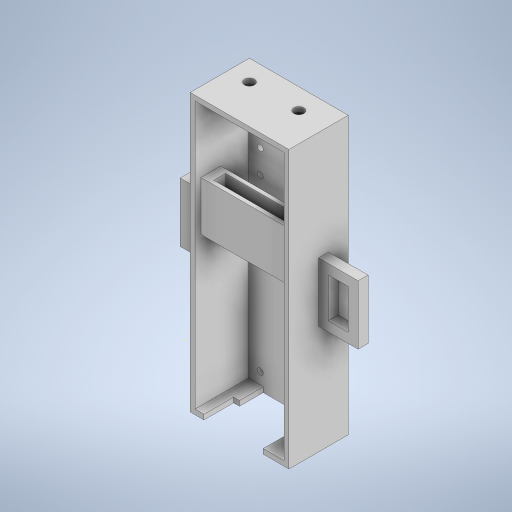
# Autodesk Inventor part: arduino mould_3r
Saved by Autodesk Inventor 2023 (Build 270158000, 158)
## iProperties
Created: 2023-05-04
Part Number: arduino mould_3r
Material: Generic
Document SubType Name: Modeling
Designer: gmami
Density: 1 g/cm^3
Appearance: Default
Author: gmami
Autodesk Inventor part; units mm, degrees
ref_plane "YZ Plane" through (0, 0, 0) normal (1, 0, 0) x (0, 1, 0)
sketch "Sketch1" plane through (0, 0, 0) normal (0, 0, 1) x (1, 0, 0)
  line L0 (33.3378, 145.104) -> (83.3378, 145.104)
  line L1 (83.3378, 145.104) -> (83.3378, 5.104)
  line L2 (83.3378, 5.104) -> (33.3378, 5.104)
  line L3 (33.3378, 5.104) -> (33.3378, 145.104)
  line L4 (33.3378, 90.104) -> (33.3378, 60.104)
  line L5 (83.3378, 90.104) -> (83.3378, 60.104)
  point P0 (0, 0)
  dimension "d0" = 140
  dimension "d1" = 50
  constraints: 12 end point, 2 parallel, 2 point on line, 1 horizontal, 1 perpendicular
  measures "d0" distance of L2.end L0.start
  measures "d1" distance of L1.end L2.end
extrude "Extrusion1" add sketch "Sketch1" along normal blind 30
sketch "Sketch2" plane through (0, 0, 30) normal (0, 0, 1) x (1, 0, 0)
  line L0 (35.8378, 142.604) -> (80.8378, 142.604)
  line L1 (80.8378, 142.604) -> (80.8378, 7.604)
  line L2 (80.8378, 7.604) -> (35.8378, 7.604)
  line L3 (35.8378, 7.604) -> (35.8378, 142.604)
  line L4 (83.3378, 145.104) -> (33.3378, 145.104) projected
  line L5 (83.3378, 5.104) -> (83.3378, 145.104) projected
  line L6 (33.3378, 5.104) -> (83.3378, 5.104) projected
  line L7 (33.3378, 145.104) -> (33.3378, 5.104) projected
  point P0 (0, 0)
  point P1 (58.3378, 142.604)
  dimension "d4" = 2.5
  dimension "d5" = 2.5
  dimension "d6" = 2.5
  dimension "d7" = 2.5
  constraints: 8 end point, 2 parallel, 1 horizontal, 1 midpoint, 1 perpendicular
  measures "d4" distance from line of L4 point (58.338, 142.604)
  measures "d5" distance between parallel lines of L5 L1
  measures "d6" distance between parallel lines of L2 L6
  measures "d7" distance between parallel lines of L3 L7
extrude "Extrusion2" cut sketch "Sketch2" against normal blind 27 contours L0 L1 L2 L3
sketch "Sketch3" plane through (33.3378, 5.104, 0) normal (0, -1, 0) x (1, 0, 0)
  line L0 (7, 30) -> (37, 30)
  line L1 (37, 30) -> (37, 15)
  line L2 (37, 15) -> (7, 15)
  line L3 (7, 15) -> (7, 30)
  line L4 (0, 0) -> (50, 0) projected
  line L5 (0, 0) -> (0, 30) projected
  line L6 (0, 30) -> (50, 30) projected
  line L7 (10, 15) -> (35, 15)
  line L8 (35, 15) -> (35, 3)
  line L9 (35, 3) -> (10, 3)
  line L10 (10, 3) -> (10, 15)
  point P0 (-33.3378, 0)
  point P1 (37, 22.5)
  point P2 (10, 9)
  dimension "d10" = 15
  dimension "d11" = 30
  dimension "d12" = 7
  dimension "d13" = 0
  dimension "d14" = 25
  dimension "d15" = 10
  dimension "d16" = 3
  constraints: 16 end point, 4 parallel, 2 horizontal, 2 midpoint, 2 perpendicular, 1 point on line
  measures "d10" distance between parallel lines of L2 L4
  measures "d11" distance from line of point (37, 22.5) L3
  measures "d12" distance between parallel lines of L3 L5
  measures "d13" distance between parallel lines of L6 L0
  measures "d14" distance between parallel lines of L8 L10
  measures "d15" distance from line of L5 point (10, 9)
  measures "d16" distance between parallel lines of L4 L9
extrude "Extrusion3" cut sketch "Sketch3" against normal blind 27
sketch "Sketch4" plane through (0, 0, 0) normal (0, 0, -1) x (-1, 0, 0)
  circle A0 centre (-74.8378, 13.604) radius 1.5
  circle A1 centre (-41.8378, 13.604) radius 1.5
  circle A2 centre (-41.8378, 99.604) radius 1.5
  circle A3 centre (-74.8378, 99.604) radius 1.5
  circle A4 centre (-41.8378, 111.604) radius 1.5
  circle A5 centre (-74.8378, 111.604) radius 1.5
  line L0 (-83.3378, 5.104) -> (-83.3378, 145.104) projected
  line L1 (-33.3378, 145.104) -> (-33.3378, 5.104) projected
  line L2 (-33.3378, 5.104) -> (-83.3378, 5.104) projected
  line L3 (-83.3378, 145.104) -> (-33.3378, 145.104) projected
  point P0 (0, 0)
  dimension "d19" = 8.5
  dimension "d20" = 8.5
  dimension "d21" = 8.5
  dimension "d22" = 8.5
  dimension "d23" = 3
  dimension "d24" = 3
  dimension "d25" = 8.5
  dimension "d26" = 8.5
  dimension "d27" = 8.5
  dimension "d28" = 8.5
  dimension "d29" = 3
  dimension "d30" = 3
  dimension "d31" = 3
  dimension "d32" = 3
  dimension "d33" = 12
  dimension "d34" = 12
  dimension "d35" = 33.5
  dimension "d36" = 33.5
  constraints: 6 centre point
  measures "d19" distance from line of A0.centre L0
  measures "d20" distance from line of L1 A1.centre
  measures "d21" distance from line of L2 A0.centre
  measures "d22" distance from line of L2 A1.centre
  measures "d23" diameter of A0
  measures "d24" diameter of A1
  measures "d25" distance from line of L1 A2.centre
  measures "d26" distance from line of L1 A4.centre
  measures "d27" distance from line of L0 A5.centre
  measures "d28" distance from line of L0 A3.centre
  measures "d29" diameter of A5
  measures "d30" diameter of A4
  measures "d31" diameter of A2
  measures "d32" diameter of A3
  measures "d33" distance of A3.centre A5.centre
  measures "d34" distance of A2.centre A4.centre
  measures "d35" distance from line of L3 A5.centre
  measures "d36" distance from line of L3 A4.centre
extrude "Extrusion4" cut sketch "Sketch4" against normal blind 27 contours A0 | A1 | A2 | A3 | A4 | A5
sketch "Sketch5" plane through (33.3378, 145.104, 0) normal (0, 1, 0) x (1, 0, 0)
  circle A0 centre (35.5, -10.5) radius 2.5
  circle A1 centre (10.5, -10.5) radius 2.5
  line L0 (50, 0) -> (50, -30) projected
  line L1 (50, 0) -> (0, 0) projected
  point P0 (-33.3378, 0)
  dimension "d39" = 5
  dimension "d40" = 5
  dimension "d41" = 25
  dimension "d42" = 14.5
  dimension "d43" = 10.5
  dimension "d44" = 10.5
  constraints: 2 centre point
  measures "d39" diameter of A0
  measures "d40" diameter of A1
  measures "d41" distance of A1.centre A0.centre
  measures "d42" distance from line of L0 A0.centre
  measures "d43" distance from line of L1 A0.centre
  measures "d44" distance from line of L1 A1.centre
extrude "Extrusion5" cut sketch "Sketch5" against normal blind 27
sketch "Sketch6" plane through (33.3378, 5.104, 0) normal (0, -1, 0) x (1, 0, 0)
  point P0 (-33.3378, 0)
ref_plane "Work Plane1" through (0, 0, 12.5) normal (0, 0, -1) x (-1, 0, 0)
sketch "Sketch7" plane through (0, 0, 12.5) normal (0, 0, -1) x (-1, 0, 0)
  line L0 (-83.3378, 5.104) -> (-83.3378, 145.104) projected
  line L1 (-83.3378, 90.104) -> (-103.3378, 90.104)
  line L2 (-103.3378, 90.104) -> (-103.3378, 60.104)
  line L3 (-103.3378, 60.104) -> (-83.3378, 60.104)
  line L4 (-83.3378, 60.104) -> (-83.3378, 90.104)
  line L5 (-83.3378, 145.104) -> (-33.3378, 145.104) projected
  line L6 (-88.3378, 65.104) -> (-98.3378, 65.104)
  line L7 (-98.3378, 65.104) -> (-98.3378, 85.104)
  line L8 (-98.3378, 85.104) -> (-88.3378, 85.104)
  line L9 (-88.3378, 85.104) -> (-88.3378, 65.104)
  line L10 (-33.3378, 145.104) -> (-33.3378, 5.104) projected
  line L11 (-13.3378, 90.104) -> (-33.3378, 90.104)
  line L12 (-33.3378, 90.104) -> (-33.3378, 60.104)
  line L13 (-33.3378, 60.104) -> (-13.3378, 60.104)
  line L14 (-13.3378, 60.104) -> (-13.3378, 90.104)
  line L15 (-18.3378, 85.104) -> (-28.3378, 85.104)
  line L16 (-28.3378, 85.104) -> (-28.3378, 65.104)
  line L17 (-28.3378, 65.104) -> (-18.3378, 65.104)
  line L18 (-18.3378, 65.104) -> (-18.3378, 85.104)
  point P0 (0, 0)
  point P1 (-93.3378, 60.104)
  dimension "d56" = 20
  dimension "d57" = 30
  dimension "d58" = 55
  dimension "d59" = 5
  dimension "d60" = 20
  dimension "d61" = 30
  dimension "d62" = 55
  dimension "d63" = 5
  constraints: 32 end point, 8 parallel, 4 perpendicular, 2 horizontal, 2 point on line, 1 midpoint, 6 other
  measures "d56" distance between parallel lines of L0 L2
  measures "d57" distance from line of L1 point (-93.338, 60.104)
  measures "d58" distance between parallel lines of L5 L1
  measures "d59" distance between parallel lines of L3 L6
  measures "d60" distance between parallel lines of L12 L14
  measures "d61" distance between parallel lines of L11 L13
  measures "d62" distance between parallel lines of L5 L11
  measures "d63" distance between parallel lines of L14 L18
extrude "Extrusion6" add sketch "Sketch7" along normal mid plane 5
ref_plane "Work Plane2" through (0, 0, 27) normal (0, 0, 1) x (1, 0, 0)
sketch "Sketch8" plane through (0, 0, 27) normal (0, 0, 1) x (1, 0, 0)
  line L0 (80.8378, 142.604) -> (80.8378, 7.604) projected
  line L1 (35.8378, 7.604) -> (35.8378, 142.604) projected
  line L2 (80.8378, 107.604) -> (35.8378, 107.604)
  line L3 (35.8378, 107.604) -> (35.8378, 82.604)
  line L4 (35.8378, 82.604) -> (80.8378, 82.604)
  line L5 (80.8378, 82.604) -> (80.8378, 107.604)
  line L6 (35.8378, 142.604) -> (80.8378, 142.604) projected
  point P0 (0, 0)
  dimension "d67" = 35
  dimension "d68" = 25
  constraints: 8 end point, 2 parallel, 2 point on line, 1 horizontal, 1 perpendicular
  measures "d67" distance between parallel lines of L6 L2
  measures "d68" distance between parallel lines of L4 L2
extrude "Extrusion7" add sketch "Sketch8" against normal blind 10 contours L0 L4 L1 L2
sketch "Sketch9" plane through (35.8378, 82.604, 27) normal (0, -1, 0) x (1, 0, 0)
  line L0 (43, -2) -> (2, -2)
  line L1 (2, -2) -> (2, -8)
  line L2 (2, -8) -> (43, -8)
  line L3 (43, -8) -> (43, -2)
  line L4 (4.5, -12) -> (4.5, 3) projected
  line L5 (0, 0) -> (45, 0) projected
  line L6 (45, -10) -> (0, -10) projected
  line L7 (0, -10) -> (0, 0) projected
  point P0 (-35.8378, -27)
  point P1 (45, 3)
  point P2 (4.5, -2)
  point P3 (4.5, -8)
  dimension "d72" = 2
  dimension "d73" = 2
  dimension "d74" = 2
  dimension "d75" = 2
  constraints: 8 end point, 2 parallel, 1 horizontal, 1 perpendicular
  measures "d72" distance between parallel lines of L5 L0
  measures "d73" distance between parallel lines of L6 L2
  measures "d74" distance from line of point (45, 3) L3
  measures "d75" distance between parallel lines of L7 L1
extrude "Extrusion8" cut sketch "Sketch9" against normal blind 27 contours L3 L2 L4 L0
body "Solid1"
